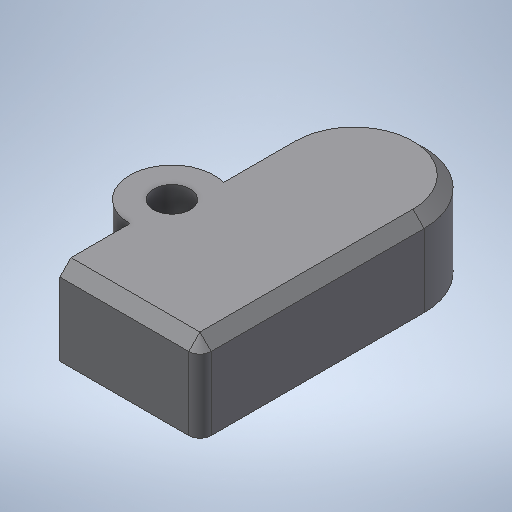
# Autodesk Inventor part: SampleComplexPart
Saved by Autodesk Inventor 2027 (Build 310192060, 192F)
## iProperties
Created: 2026-06-17
Part Number: SampleComplexPart
Material: Generisch
Document SubType Name: Modeling
Designer: tobia
Density: 1 g/cm^3
Appearance: Vorgabe
Author: tobia
Autodesk Inventor part; units mm, degrees
ref_plane "YZ Plane" through (0, 0, 0) normal (1, 0, 0) x (0, 1, 0)
ref_plane "XZ Plane" through (0, 0, 0) normal (0, 1, 0) x (-1, 0, 0)
ref_plane "XY Plane" through (0, 0, 0) normal (0, 0, 1) x (1, 0, 0)
sketch "Sketch1" plane through (0, 0, 0) normal (0, 1, 0) x (-1, 0, 0)
  line L0 (-12.5, -20) -> (12.5, -20)
  line L1 (12.5, -20) -> (12.5, 20)
  line L2 (12.5, 20) -> (-12.5, 20)
  line L3 (-12.5, 20) -> (-12.5, -20)
  line L4 (-12.5, -20) -> (12.5, 20) construction
  line L5 (12.5, -20) -> (-12.5, 20) construction
  circle A0 centre (0, -20) radius 12.5
  circle A1 centre (12.5, 0) radius 7.5
  point P0 (0, 0)
  point P1 (12.5, -7.5)
  point P2 (12.5, 7.5)
  dimension "d0" = 25
  dimension "d1" = 40
  dimension "d2" = 15
  constraints: 12 end point, 4 midpoint, 2 parallel, 1 centre point, 1 horizontal, 1 perpendicular, 3 other
  measures "d0" distance of L2.end L1.end
  measures "d1" distance of L1.end L0.end
  measures "d2" diameter of A1
extrude "Extrusion1" add sketch "Sketch1" along normal blind 15
fillet "Fillet1" radius 2 1 edges at (12.5, 7.5, 20)
chamfer "Chamfer1" distance 2 angle 45 5 edges at (-1, 15, 20) (11.9142, 15, 19.4142) (12.5, 15, -1) (0, 15, -32.5) (-12.5, 15, -13.75)
sketch "Sketch2" plane through (0, 15, 0) normal (0, 1, 0) x (1, 0, 0)
  arc A0 (-10.5, 7.2284) -> (-12.5, -7.5) centre (-12.5, 0) ccw projected
  point P0 (0, 0)
  constraints: 1 coincident
hole "Hole1" at (-12.5, 15, 0) direction (0, -1, 0) diameter 6.5 end through all
equation "\"d3\" = d2"
body "Solid1"
